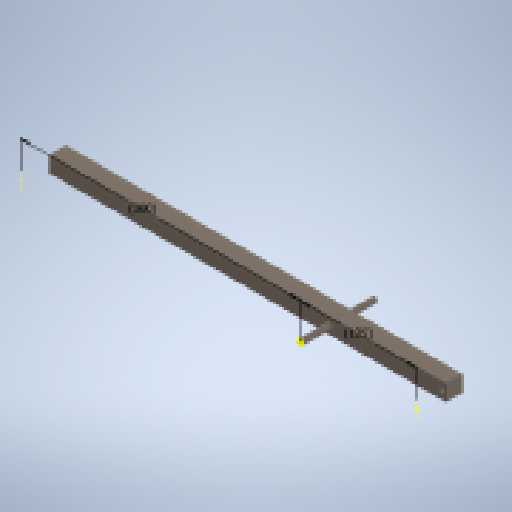
# Autodesk Inventor part: Long Arm
Saved by Autodesk Inventor 2025.2 (Build 292293000, 293)
## iProperties
Created: 2025-02-17
Part Number: Long Arm
Material: Generic
Document SubType Name: Modeling
Designer: baolo
Density: 1 g/cm^3
Appearance: Walnut
Mass: 138.128 g
Surface Area: 291.717 cm^2
Volume: 138.128 cm^3
LongArmLen: 0.300 m
Author: baolo
Autodesk Inventor part; units mm, degrees
ref_plane "YZ Plane" through (0, 0, 0) normal (1, 0, 0) x (0, 1, 0)
ref_plane "XZ Plane" through (0, 0, 0) normal (0, 1, 0) x (-1, 0, 0)
sketch "Sketch1" plane through (0, 0, 0) normal (1, 0, 0) x (0, 1, 0)
  line L0 (8.7312, 8.7312) -> (-8.7312, 8.7312)
  line L1 (-8.7312, 8.7312) -> (-8.7313, -8.7313)
  line L2 (-8.7313, -8.7313) -> (8.7312, -8.7313)
  line L3 (8.7312, -8.7313) -> (8.7312, 8.7312)
  line L4 (8.7312, 8.7312) -> (-8.7313, -8.7313) construction
  line L5 (-8.7312, 8.7312) -> (8.7312, -8.7313) construction
  point P0 (0, 0)
  point P1 (0, 0)
  dimension "d9" = 17.4625
  dimension "d10" = 17.4625
  constraints: 12 end point, 2 parallel, 1 coincident, 1 horizontal, 1 midpoint, 1 perpendicular
  measures "d9" distance of L2.end L1.end
  measures "d10" distance of L1.end L0.end
extrude "Extrusion1" add sketch "Sketch1" against normal blind 425
ref_plane "Work Plane2" through (0, 0, 10) normal (0, 0, 1) x (1, 0, 0)
sketch "Sketch2" plane through (0, 0, 0) normal (0, 0, 1) x (1, 0, 0)
  circle A0 centre (-125, 0) radius 3.175
  line L0 (0, 8.7312) -> (0, -8.7312) construction
  line L1 (-425, 8.7312) -> (-425, -8.7313) construction
  point P0 (0, 0)
  dimension "d7" = 6.35
  dimension "d11" = 300
  constraints: 1 centre point, 1 coincident, 1 horizontal alignment, 1 midpoint
  measures "d7" diameter of A0
  measures "d11" distance from line of point (-125, 0) L1
extrude "Extrusion2" add sketch "Sketch2" along normal mid plane 80
sketch "Sketch4" plane through (0, -8.7312, 8.7312) normal (0, 0, 1) x (1, 0, 0)
  circle A0 centre (-125, 8.7312) radius 3.175 construction
  point P0 (0, 8.7312)
  point P1 (-5, 8.7312)
  dimension "d14" = 120
  constraints: 1 horizontal alignment
  measures "d14" distance of A0.centre point (-5, 8.731)
hole "Hole1" at (-5, 0, 8.7312) direction (0, 0, -1) diameter 5 end through all
sketch "Sketch3" plane through (-125, 0, 40) normal (0, 0, 1) x (1, 0, 0)
  circle A0 centre (0, 0) radius 3.175 projected
  line L0 (-300, -8.7312) -> (-300, 8.7312) construction
  line L1 (125, 8.7312) -> (125, -8.7312) construction
  point P0 (125, 0)
  dimension "d12" = 300
  dimension "d13" = 125
  measures "d12" distance from line of L0 A0.centre
  measures "d13" distance from line of L1 A0.centre
equation "\"d11\" = LongArmLen"
equation "\"d14\" = ShortArmLen"
equation "\"LongArmLen\" = 300"
equation "\"ShortArmLen\" = 120"
body "Solid1"
